Autodesk Inventor part; units mm, degrees
(part 2 of 2)
sketch "Эскиз6" plane through (0, 0, 0) normal (0, 0, -1) x (-1, 0, 0)
  line L0 (-53, 15.6179) -> (-25.3405, 4.0009) projected
  line L1 (-25.3405, 4.0009) -> (-8.0842, -5.3702) projected
  line L2 (-7.9523, -5.3473) -> (-8.0842, -5.3702) projected
  line L3 (-7.789, -5.3433) -> (-7.9523, -5.3473) projected
  line L4 (-7.444, -5.4468) -> (-7.789, -5.3433) projected
  line L5 (-6.7921, -5.8052) -> (-7.444, -5.4468) projected
  line L6 (-6.1197, -6.1235) -> (-6.7921, -5.8052) projected
  line L7 (-5.8336, -6.3424) -> (-6.1197, -6.1235) projected
  line L8 (-5.7412, -6.4771) -> (-5.8336, -6.3424) projected
  line L9 (-5.6824, -6.5974) -> (-5.7412, -6.4771) projected
  line L10 (-5.6419, -6.7101) -> (-5.6824, -6.5974) projected
  line L11 (-5.6135, -6.8178) -> (-5.6419, -6.7101) projected
  line L12 (-5.5818, -7.0232) -> (-5.6135, -6.8178) projected
  line L13 (-5.5741, -7.2193) -> (-5.5818, -7.0232) projected
  line L14 (-5.5841, -7.4089) -> (-5.5741, -7.2193) projected
  line L15 (-5.6083, -7.5933) -> (-5.5841, -7.4089) projected
  line L16 (-5.691, -7.9502) -> (-5.6083, -7.5933) projected
  line L17 (-5.802, -8.2972) -> (-5.691, -7.9502) projected
  line L18 (-5.8532, -8.6645) -> (-5.802, -8.2972) projected
  line L19 (-5.864, -9.0449) -> (-5.8532, -8.6645) projected
  line L20 (-5.8437, -9.4343) -> (-5.864, -9.0449) projected
  line L21 (-5.7962, -9.8308) -> (-5.8437, -9.4343) projected
  line L22 (-5.7233, -10.2331) -> (-5.7962, -9.8308) projected
  line L23 (-5.6263, -10.6399) -> (-5.7233, -10.2331) projected
  line L24 (-5.5062, -11.0504) -> (-5.6263, -10.6399) projected
  line L25 (-5.3633, -11.4634) -> (-5.5062, -11.0504) projected
  line L26 (-5.1983, -11.8783) -> (-5.3633, -11.4634) projected
  line L27 (-5.0602, -12.1901) -> (-5.1983, -11.8783) projected
  line L28 (-2.9375, -12.5288) -> (-5.0602, -12.1901) projected
  line L29 (-2.7092, -12.2754) -> (-2.9375, -12.5288) projected
  line L30 (-2.4233, -11.9325) -> (-2.7092, -12.2754) projected
  line L31 (-2.159, -11.5843) -> (-2.4233, -11.9325) projected
  line L32 (-1.9171, -11.2317) -> (-2.159, -11.5843) projected
  line L33 (-1.6983, -10.8752) -> (-1.9171, -11.2317) projected
  line L34 (-1.5039, -10.5156) -> (-1.6983, -10.8752) projected
  line L35 (-1.3353, -10.1535) -> (-1.5039, -10.5156) projected
  line L36 (-1.1949, -9.7897) -> (-1.3353, -10.1535) projected
  line L37 (-1.0869, -9.4249) -> (-1.1949, -9.7897) projected
  line L38 (-1.0212, -9.0599) -> (-1.0869, -9.4249) projected
  line L39 (-1.0187, -8.6955) -> (-1.0212, -9.0599) projected
  line L40 (-0.9863, -8.3307) -> (-1.0187, -8.6955) projected
  line L41 (-0.9519, -8.1479) -> (-0.9863, -8.3307) projected
  line L42 (-0.9024, -7.9646) -> (-0.9519, -8.1479) projected
  line L43 (-0.834, -7.7806) -> (-0.9024, -7.9646) projected
  line L44 (-0.74, -7.5953) -> (-0.834, -7.7806) projected
  line L45 (-0.6795, -7.5017) -> (-0.74, -7.5953) projected
  line L46 (-0.6059, -7.4072) -> (-0.6795, -7.5017) projected
  line L47 (-0.5127, -7.3112) -> (-0.6059, -7.4072) projected
  line L48 (-0.3829, -7.2119) -> (-0.5127, -7.3112) projected
  line L49 (-0.0429, -7.0929) -> (-0.3829, -7.2119) projected
  line L50 (0.6951, -6.9997) -> (-0.0429, -7.0929) projected
  line L51 (1.4262, -6.8619) -> (0.6951, -6.9997) projected
  line L52 (1.7863, -6.8709) -> (1.4262, -6.8619) projected
  line L53 (1.9402, -6.9255) -> (1.7863, -6.8709) projected
  line L54 (2.0585, -6.9883) -> (1.9402, -6.9255) projected
  line L55 (2.1575, -7.0556) -> (2.0585, -6.9883) projected
  line L56 (2.2438, -7.1261) -> (2.1575, -7.0556) projected
  line L57 (2.3901, -7.2737) -> (2.2438, -7.1261) projected
  line L58 (2.5117, -7.4278) -> (2.3901, -7.2737) projected
  line L59 (2.615, -7.5871) -> (2.5117, -7.4278) projected
  line L60 (2.7039, -7.7505) -> (2.615, -7.5871) projected
  line L61 (2.8467, -8.0877) -> (2.7039, -7.7505) projected
  line L62 (2.9609, -8.4338) -> (2.8467, -8.0877) projected
  line L63 (3.1354, -8.7611) -> (2.9609, -8.4338) projected
  line L64 (3.3502, -9.0751) -> (3.1354, -8.7611) projected
  line L65 (3.5955, -9.3782) -> (3.3502, -9.0751) projected
  line L66 (3.867, -9.6711) -> (3.5955, -9.3782) projected
  line L67 (4.1624, -9.9537) -> (3.867, -9.6711) projected
  line L68 (4.48, -10.2258) -> (4.1624, -9.9537) projected
  line L69 (4.8185, -10.4872) -> (4.48, -10.2258) projected
  line L70 (5.1768, -10.7375) -> (4.8185, -10.4872) projected
  line L71 (5.5542, -10.9761) -> (5.1768, -10.7375) projected
  line L72 (5.8492, -11.1472) -> (5.5542, -10.9761) projected
  line L73 (7.7656, -10.1735) -> (5.8492, -11.1472) projected
  line L74 (7.8013, -9.8343) -> (7.7656, -10.1735) projected
  line L75 (7.8311, -9.3888) -> (7.8013, -9.8343) projected
  line L76 (7.8403, -8.9518) -> (7.8311, -9.3888) projected
  line L77 (7.8287, -8.5243) -> (7.8403, -8.9518) projected
  line L78 (7.7961, -8.1074) -> (7.8287, -8.5243) projected
  line L79 (7.742, -7.7022) -> (7.7961, -8.1074) projected
  line L80 (7.6656, -7.3102) -> (7.742, -7.7022) projected
  line L81 (7.5654, -6.9333) -> (7.6656, -7.3102) projected
  line L82 (7.4384, -6.5746) -> (7.5654, -6.9333) projected
  line L83 (7.2769, -6.2407) -> (7.4384, -6.5746) projected
  line L84 (7.0647, -5.9445) -> (7.2769, -6.2407) projected
  line L85 (6.8765, -5.6303) -> (7.0647, -5.9445) projected
  line L86 (6.7969, -5.4622) -> (6.8765, -5.6303) projected
  line L87 (6.7292, -5.2848) -> (6.7969, -5.4622) projected
  line L88 (6.6764, -5.0958) -> (6.7292, -5.2848) projected
  line L89 (6.6435, -4.8906) -> (6.6764, -5.0958) projected
  line L90 (6.6374, -4.7793) -> (6.6435, -4.8906) projected
  line L91 (6.6415, -4.6596) -> (6.6374, -4.7793) projected
  line L92 (6.6604, -4.5271) -> (6.6415, -4.6596) projected
  line L93 (6.7071, -4.3705) -> (6.6604, -4.5271) projected
  line L94 (6.9122, -4.0744) -> (6.7071, -4.3705) projected
  line L95 (7.4545, -3.5652) -> (6.9122, -4.0744) projected
  line L96 (7.9649, -3.024) -> (7.4545, -3.5652) projected
  line L97 (8.2615, -2.8196) -> (7.9649, -3.024) projected
  line L98 (8.4182, -2.7733) -> (8.2615, -2.8196) projected
  line L99 (8.5508, -2.7546) -> (8.4182, -2.7733) projected
  line L100 (8.6705, -2.7509) -> (8.5508, -2.7546) projected
  line L101 (8.7817, -2.7571) -> (8.6705, -2.7509) projected
  line L102 (8.9868, -2.7905) -> (8.7817, -2.7571) projected
  line L103 (9.1758, -2.8438) -> (8.9868, -2.7905) projected
  line L104 (9.353, -2.9118) -> (9.1758, -2.8438) projected
  line L105 (9.5209, -2.9918) -> (9.353, -2.9118) projected
  line L106 (9.8347, -3.1808) -> (9.5209, -2.9918) projected
  line L107 (10.1304, -3.3936) -> (9.8347, -3.1808) projected
  line L108 (10.464, -3.5558) -> (10.1304, -3.3936) projected
  line L109 (10.8224, -3.6836) -> (10.464, -3.5558) projected
  line L110 (11.199, -3.7847) -> (10.8224, -3.6836) projected
  line L111 (11.5908, -3.862) -> (11.199, -3.7847) projected
  line L112 (11.9959, -3.917) -> (11.5908, -3.862) projected
  line L113 (12.4128, -3.9505) -> (11.9959, -3.917) projected
  line L114 (12.8403, -3.963) -> (12.4128, -3.9505) projected
  line L115 (13.2773, -3.9548) -> (12.8403, -3.963) projected
  line L116 (13.7228, -3.9261) -> (13.2773, -3.9548) projected
  line L117 (14.0621, -3.891) -> (13.7228, -3.9261) projected
  line L118 (15.0401, -1.9769) -> (14.0621, -3.891) projected
  line L119 (14.8697, -1.6815) -> (15.0401, -1.9769) projected
  line L120 (14.6319, -1.3036) -> (14.8697, -1.6815) projected
  line L121 (14.3824, -0.9447) -> (14.6319, -1.3036) projected
  line L122 (14.1218, -0.6056) -> (14.3824, -0.9447) projected
  line L123 (13.8504, -0.2874) -> (14.1218, -0.6056) projected
  line L124 (13.5684, 0.0086) -> (13.8504, -0.2874) projected
  line L125 (13.2762, 0.2808) -> (13.5684, 0.0086) projected
  line L126 (12.9736, 0.5268) -> (13.2762, 0.2808) projected
  line L127 (12.66, 0.7423) -> (12.9736, 0.5268) projected
  line L128 (12.3332, 0.9175) -> (12.66, 0.7423) projected
  line L129 (11.9874, 1.0325) -> (12.3332, 0.9175) projected
  line L130 (11.6504, 1.1761) -> (11.9874, 1.0325) projected
  line L131 (11.4872, 1.2653) -> (11.6504, 1.1761) projected
  line L132 (11.3282, 1.369) -> (11.4872, 1.2653) projected
  line L133 (11.1743, 1.4909) -> (11.3282, 1.369) projected
  line L134 (11.0271, 1.6375) -> (11.1743, 1.4909) projected
  line L135 (10.9568, 1.724) -> (11.0271, 1.6375) projected
  line L136 (10.8897, 1.8232) -> (10.9568, 1.724) projected
  line L137 (10.8272, 1.9416) -> (10.8897, 1.8232) projected
  line L138 (10.7729, 2.0956) -> (10.8272, 1.9416) projected
  line L139 (10.7647, 2.4558) -> (10.7729, 2.0956) projected
  line L140 (10.9042, 3.1865) -> (10.7647, 2.4558) projected
  line L141 (10.999, 3.9243) -> (10.9042, 3.1865) projected
  line L142 (11.1188, 4.264) -> (10.999, 3.9243) projected
  line L143 (11.2183, 4.3936) -> (11.1188, 4.264) projected
  line L144 (11.3146, 4.4866) -> (11.2183, 4.3936) projected
  line L145 (11.4093, 4.56) -> (11.3146, 4.4866) projected
  line L146 (11.5029, 4.6203) -> (11.4093, 4.56) projected
  line L147 (11.6885, 4.7139) -> (11.5029, 4.6203) projected
  line L148 (11.8727, 4.7818) -> (11.6885, 4.7139) projected
  line L149 (12.056, 4.8309) -> (11.8727, 4.7818) projected
  line L150 (12.2389, 4.8649) -> (12.056, 4.8309) projected
  line L151 (12.6038, 4.8965) -> (12.2389, 4.8649) projected
  line L152 (12.9682, 4.8982) -> (12.6038, 4.8965) projected
  line L153 (13.3334, 4.963) -> (12.9682, 4.8982) projected
  line L154 (13.6984, 5.0703) -> (13.3334, 4.963) projected
  line L155 (14.0625, 5.2099) -> (13.6984, 5.0703) projected
  line L156 (14.425, 5.3776) -> (14.0625, 5.2099) projected
  line L157 (14.785, 5.5713) -> (14.425, 5.3776) projected
  line L158 (15.142, 5.7892) -> (14.785, 5.5713) projected
  line L159 (15.4952, 6.0303) -> (15.142, 5.7892) projected
  line L160 (15.8439, 6.2938) -> (15.4952, 6.0303) projected
  line L161 (16.1875, 6.579) -> (15.8439, 6.2938) projected
  line L162 (16.4414, 6.8067) -> (16.1875, 6.579) projected
  line L163 (16.1075, 8.9301) -> (16.4414, 6.8067) projected
  line L164 (15.796, 9.069) -> (16.1075, 8.9301) projected
  line L165 (15.3815, 9.2349) -> (15.796, 9.069) projected
  line L166 (14.9687, 9.3787) -> (15.3815, 9.2349) projected
  line L167 (14.5586, 9.4998) -> (14.9687, 9.3787) projected
  line L168 (14.1519, 9.5976) -> (14.5586, 9.4998) projected
  line L169 (13.7498, 9.6714) -> (14.1519, 9.5976) projected
  line L170 (13.3534, 9.7199) -> (13.7498, 9.6714) projected
  line L171 (12.964, 9.741) -> (13.3534, 9.7199) projected
  line L172 (12.5837, 9.731) -> (12.964, 9.741) projected
  line L173 (12.2162, 9.6807) -> (12.5837, 9.731) projected
  line L174 (11.8689, 9.5704) -> (12.2162, 9.6807) projected
  line L175 (11.5119, 9.4885) -> (11.8689, 9.5704) projected
  line L176 (11.3274, 9.4648) -> (11.5119, 9.4885) projected
  line L177 (11.1379, 9.4552) -> (11.3274, 9.4648) projected
  line L178 (10.9417, 9.4634) -> (11.1379, 9.4552) projected
  line L179 (10.7364, 9.4955) -> (10.9417, 9.4634) projected
  line L180 (10.6287, 9.5241) -> (10.7364, 9.4955) projected
  line L181 (10.5161, 9.5649) -> (10.6287, 9.5241) projected
  line L182 (10.3959, 9.6239) -> (10.5161, 9.5649) projected
  line L183 (10.2615, 9.7167) -> (10.3959, 9.6239) projected
  line L184 (10.0432, 10.0032) -> (10.2615, 9.7167) projected
  line L185 (9.7265, 10.6764) -> (10.0432, 10.0032) projected
  line L186 (9.3696, 11.329) -> (9.7265, 10.6764) projected
  line L187 (9.2668, 11.6743) -> (9.3696, 11.329) projected
  line L188 (9.2712, 11.8376) -> (9.2668, 11.6743) projected
  line L189 (9.2943, 11.9695) -> (9.2712, 11.8376) projected
  line L190 (9.3278, 12.0845) -> (9.2943, 11.9695) projected
  line L191 (9.3681, 12.1883) -> (9.3278, 12.0845) projected
  line L192 (9.4633, 12.3731) -> (9.3681, 12.1883) projected
  line L193 (9.5723, 12.5363) -> (9.4633, 12.3731) projected
  line L194 (9.6918, 12.6838) -> (9.5723, 12.5363) projected
  line L195 (9.8198, 12.8188) -> (9.6918, 12.6838) projected
  line L196 (10.0964, 13.0589) -> (9.8198, 12.8188) projected
  line L197 (10.3902, 13.2744) -> (10.0964, 13.0589) projected
  line L198 (10.6476, 13.5415) -> (10.3902, 13.2744) projected
  line L199 (10.8798, 13.8428) -> (10.6476, 13.5415) projected
  line L200 (11.0924, 14.1698) -> (10.8798, 13.8428) projected
  line L201 (11.1891, 14.3431) -> (11.0924, 14.1698) projected
  arc A0 (11.1891, 14.3431) -> (-16.1963, 14.3431) centre (-2.5036, -3.8906) ccw projected
  arc A1 (-25.3405, 9.161) -> (-16.1963, 14.3431) centre (-40.8164, 47.1281) ccw projected
  line L202 (-25.3405, 9.161) -> (-53, 20.778) projected
  line L203 (-53, 20.778) -> (-57, 20.778) projected
  line L204 (-57, 20.778) -> (-57, 17.5182) projected
  line L205 (-57, 17.5182) -> (-76.2555, 1.8259) projected
  line L206 (-76.2555, 1.8259) -> (-73.7286, -1.2748) projected
  line L207 (-73.7286, -1.2748) -> (-57, 12.3581) projected
  line L208 (-57, 12.3581) -> (-57, -9) projected
  line L209 (-57, -9) -> (-53, -9) projected
  line L210 (-53, -9) -> (-53, 15.6179) projected
  circle A2 centre (-8.3767, 1.5633) radius 1.6 projected
  circle A3 centre (2.3455, -2.0471) radius 1.6 projected
  circle A4 centre (5.9559, 8.675) radius 1.6 projected
  circle A5 centre (-4.7663, 12.2855) radius 1.6 projected
  circle A6 centre (-1.2104, 5.1192) radius 2.5 projected
  line L211 (-57, 17.5182) -> (-57, 12.3581)
  point P0 (0, 0)
  constraints: 2 end point, 1 collinear
extrude "Выдавливание6" cut sketch "Эскиз6" against normal blind 10 contours L207 L206 L205 L211
sketch "Эскиз7" plane through (0, 0, 5) normal (0, 0, 1) x (1, 0, 0)
  line L0 (39.5581, 1.9289) -> (53.904, -11.9897) projected
  line L1 (39.5581, 1.9289) -> (53.904, -11.9897) construction
  line L2 (71.9316, -0.8693) -> (40.2367, -32.4918) construction
  line L3 (71.9316, -0.8693) -> (71.9317, -0.7909) construction
  line L4 (71.9317, -0.7909) -> (40.1893, -0.7429) construction
  line L5 (40.1893, -0.7429) -> (40.1583, -32.5308) construction
  ellipse E0 centre (40.323, 96.1032) end of major axis (40.1583, -32.5308) minor radius 3.174 (40.1583, -32.5308) -> (40.2367, -32.4918) ccw construction
  line L6 (71.9495, -32.6204) -> (72.0099, -0.8302) construction
  ellipse E1 centre (71.7261, -129.4732) end of major axis (71.4423, -258.1162) minor radius 3.1711 (72.0099, -0.8302) -> (71.9316, -0.8693) ccw construction
  line L7 (71.9316, -0.8693) -> (40.2367, -32.4918) construction
  line L8 (40.2367, -32.4918) -> (40.2366, -32.5701) construction
  line L9 (40.2366, -32.5701) -> (71.9495, -32.6204) construction
  line L10 (61.1948, -58.9491) -> (61.3584, -29.5225) projected
  line L11 (61.3584, -29.5225) -> (54.845, -29.4863) projected
  line L12 (54.845, -29.4863) -> (43.8928, -40.4135) projected
  line L13 (43.8928, -40.4135) -> (39.1927, -45.5003) projected
  line L14 (39.1927, -45.5003) -> (23.9385, -36.7753) projected
  line L15 (9.9184, -17.7195) -> (23.9385, -36.7753) projected
  line L16 (9.9184, -17.7195) -> (9.6501, -17.5929) projected
  line L17 (9.4478, -17.7158) -> (9.6501, -17.5929) projected
  line L18 (9.1396, -17.9389) -> (9.4478, -17.7158) projected
  line L19 (8.8648, -18.188) -> (9.1396, -17.9389) projected
  line L20 (8.6405, -18.4751) -> (8.8648, -18.188) projected
  line L21 (8.3922, -18.7444) -> (8.6405, -18.4751) projected
  line L22 (8.2533, -18.8682) -> (8.3922, -18.7444) projected
  line L23 (8.1023, -18.9831) -> (8.2533, -18.8682) projected
  line L24 (7.9358, -19.0872) -> (8.1023, -18.9831) projected
  line L25 (7.7483, -19.1767) -> (7.9358, -19.0872) projected
  line L26 (7.6432, -19.2139) -> (7.7483, -19.1767) projected
  line L27 (7.5273, -19.2438) -> (7.6432, -19.2139) projected
  line L28 (7.3948, -19.263) -> (7.5273, -19.2438) projected
  line L29 (7.2314, -19.2624) -> (7.3948, -19.263) projected
  line L30 (6.8894, -19.1492) -> (7.2314, -19.2624) projected
  line L31 (6.2479, -18.7726) -> (6.8894, -19.1492) projected
  line L32 (5.5847, -18.4357) -> (6.2479, -18.7726) projected
  line L33 (5.3049, -18.2088) -> (5.5847, -18.4357) projected
  line L34 (5.2162, -18.0716) -> (5.3049, -18.2088) projected
  line L35 (5.1609, -17.9496) -> (5.2162, -18.0716) projected
  line L36 (5.1235, -17.8359) -> (5.1609, -17.9496) projected
  line L37 (5.0982, -17.7274) -> (5.1235, -17.8359) projected
  line L38 (5.0723, -17.5212) -> (5.0982, -17.7274) projected
  line L39 (5.0701, -17.3249) -> (5.0723, -17.5212) projected
  line L40 (5.0854, -17.1357) -> (5.0701, -17.3249) projected
  line L41 (5.1147, -16.952) -> (5.0854, -17.1357) projected
  line L42 (5.2074, -16.5976) -> (5.1147, -16.952) projected
  line L43 (5.3282, -16.2538) -> (5.2074, -16.5976) projected
  line L44 (5.3896, -15.8881) -> (5.3282, -16.2538) projected
  line L45 (5.4111, -15.5082) -> (5.3896, -15.8881) projected
  line L46 (5.4018, -15.1184) -> (5.4111, -15.5082) projected
  line L47 (5.3654, -14.7206) -> (5.4018, -15.1184) projected
  line L48 (5.3039, -14.3165) -> (5.3654, -14.7206) projected
  line L49 (5.2184, -13.9071) -> (5.3039, -14.3165) projected
  line L50 (5.1098, -13.4935) -> (5.2184, -13.9071) projected
  line L51 (4.9786, -13.0765) -> (5.1098, -13.4935) projected
  line L52 (4.8253, -12.6572) -> (4.9786, -13.0765) projected
  line L53 (4.696, -12.3416) -> (4.8253, -12.6572) projected
  line L54 (2.5836, -11.9435) -> (4.696, -12.3416) projected
  line L55 (2.3483, -12.1904) -> (2.5836, -11.9435) projected
  line L56 (2.0529, -12.5251) -> (2.3483, -12.1904) projected
  line L57 (1.7789, -12.8657) -> (2.0529, -12.5251) projected
  line L58 (1.5272, -13.2114) -> (1.7789, -12.8657) projected
  line L59 (1.2985, -13.5616) -> (1.5272, -13.2114) projected
  line L60 (1.0941, -13.9156) -> (1.2985, -13.5616) projected
  line L61 (0.9154, -14.2728) -> (1.0941, -13.9156) projected
  line L62 (0.7648, -14.6325) -> (0.9154, -14.2728) projected
  line L63 (0.6465, -14.9941) -> (0.7648, -14.6325) projected
  line L64 (0.5707, -15.3572) -> (0.6465, -14.9941) projected
  line L65 (0.558, -15.7213) -> (0.5707, -15.3572) projected
  line L66 (0.5153, -16.0851) -> (0.558, -15.7213) projected
  line L67 (0.4758, -16.2669) -> (0.5153, -16.0851) projected
  line L68 (0.4212, -16.4487) -> (0.4758, -16.2669) projected
  line L69 (0.3476, -16.6307) -> (0.4212, -16.4487) projected
  line L70 (0.2485, -16.8133) -> (0.3476, -16.6307) projected
  line L71 (0.1854, -16.9051) -> (0.2485, -16.8133) projected
  line L72 (0.1092, -16.9975) -> (0.1854, -16.9051) projected
  line L73 (0.0132, -17.0909) -> (0.1092, -16.9975) projected
  line L74 (-0.1193, -17.1865) -> (0.0132, -17.0909) projected
  line L75 (-0.4625, -17.2959) -> (-0.1193, -17.1865) projected
  line L76 (-1.2028, -17.3684) -> (-0.4625, -17.2959) projected
  line L77 (-1.9374, -17.4856) -> (-1.2028, -17.3684) projected
  line L78 (-2.2972, -17.4665) -> (-1.9374, -17.4856) projected
  line L79 (-2.4495, -17.4076) -> (-2.2972, -17.4665) projected
  line L80 (-2.566, -17.3415) -> (-2.4495, -17.4076) projected
  line L81 (-2.6631, -17.2714) -> (-2.566, -17.3415) projected
  line L82 (-2.7474, -17.1985) -> (-2.6631, -17.2714) projected
  line L83 (-2.8895, -17.0469) -> (-2.7474, -17.1985) projected
  line L84 (-3.0066, -16.8894) -> (-2.8895, -17.0469) projected
  line L85 (-3.1055, -16.7273) -> (-3.0066, -16.8894) projected
  line L86 (-3.1897, -16.5615) -> (-3.1055, -16.7273) projected
  line L87 (-3.323, -16.2203) -> (-3.1897, -16.5615) projected
  line L88 (-3.4274, -15.8712) -> (-3.323, -16.2203) projected
  line L89 (-3.5927, -15.5392) -> (-3.4274, -15.8712) projected
  line L90 (-3.7986, -15.2192) -> (-3.5927, -15.5392) projected
  line L91 (-4.0352, -14.9093) -> (-3.7986, -15.2192) projected
  line L92 (-4.2985, -14.6089) -> (-4.0352, -14.9093) projected
  line L93 (-4.5858, -14.3182) -> (-4.2985, -14.6089) projected
  line L94 (-4.8956, -14.0372) -> (-4.5858, -14.3182) projected
  line L95 (-5.2266, -13.7664) -> (-4.8956, -14.0372) projected
  line L96 (-5.5778, -13.5062) -> (-5.2266, -13.7664) projected
  line L97 (-5.9483, -13.2571) -> (-5.5778, -13.5062) projected
  line L98 (-6.2384, -13.0778) -> (-5.9483, -13.2571) projected
  line L99 (-8.1813, -13.9973) -> (-6.2384, -13.0778) projected
  line L100 (-8.2266, -14.3353) -> (-8.1813, -13.9973) projected
  line L101 (-8.2689, -14.7798) -> (-8.2266, -14.3353) projected
  line L102 (-8.2903, -15.2163) -> (-8.2689, -14.7798) projected
  line L103 (-8.2908, -15.644) -> (-8.2903, -15.2163) projected
  line L104 (-8.2699, -16.0617) -> (-8.2908, -15.644) projected
  line L105 (-8.2272, -16.4683) -> (-8.2699, -16.0617) projected
  line L106 (-8.1619, -16.8623) -> (-8.2272, -16.4683) projected
  line L107 (-8.0722, -17.2418) -> (-8.1619, -16.8623) projected
  line L108 (-7.9554, -17.6039) -> (-8.0722, -17.2418) projected
  line L109 (-7.8034, -17.9422) -> (-7.9554, -17.6039) projected
  line L110 (-7.5996, -18.2443) -> (-7.8034, -17.9422) projected
  line L111 (-7.4203, -18.5636) -> (-7.5996, -18.2443) projected
  line L112 (-7.3454, -18.7339) -> (-7.4203, -18.5636) projected
  line L113 (-7.2827, -18.9131) -> (-7.3454, -18.7339) projected
  line L114 (-7.2352, -19.1036) -> (-7.2827, -18.9131) projected
  line L115 (-7.2081, -19.3096) -> (-7.2352, -19.1036) projected
  line L116 (-7.2052, -19.421) -> (-7.2081, -19.3096) projected
  line L117 (-7.2126, -19.5405) -> (-7.2052, -19.421) projected
  line L118 (-7.2353, -19.6725) -> (-7.2126, -19.5405) projected
  line L119 (-7.2863, -19.8277) -> (-7.2353, -19.6725) projected
  line L120 (-7.4996, -20.1179) -> (-7.2863, -19.8277) projected
  line L121 (-8.056, -20.6117) -> (-7.4996, -20.1179) projected
  line L122 (-8.5814, -21.1383) -> (-8.056, -20.6117) projected
  line L123 (-8.8836, -21.3343) -> (-8.5814, -21.1383) projected
  line L124 (-9.0415, -21.3762) -> (-8.8836, -21.3343) projected
  line L125 (-9.1746, -21.3912) -> (-9.0415, -21.3762) projected
  line L126 (-9.2944, -21.3915) -> (-9.1746, -21.3912) projected
  line L127 (-9.4054, -21.3821) -> (-9.2944, -21.3915) projected
  line L128 (-9.6095, -21.343) -> (-9.4054, -21.3821) projected
  line L129 (-9.7969, -21.2845) -> (-9.6095, -21.343) projected
  line L130 (-9.9721, -21.2114) -> (-9.7969, -21.2845) projected
  line L131 (-10.1377, -21.1268) -> (-9.9721, -21.2114) projected
  line L132 (-10.4461, -20.9291) -> (-10.1377, -21.1268) projected
  line L133 (-10.7357, -20.708) -> (-10.4461, -20.9291) projected
  line L134 (-11.0646, -20.5366) -> (-10.7357, -20.708) projected
  line L135 (-11.4192, -20.3987) -> (-11.0646, -20.5366) projected
  line L136 (-11.7929, -20.2871) -> (-11.4192, -20.3987) projected
  line L137 (-12.1824, -20.1988) -> (-11.7929, -20.2871) projected
  line L138 (-12.5858, -20.1325) -> (-12.1824, -20.1988) projected
  line L139 (-13.0015, -20.0873) -> (-12.5858, -20.1325) projected
  line L140 (-13.4285, -20.0628) -> (-13.0015, -20.0873) projected
  line L141 (-13.8655, -20.0587) -> (-13.4285, -20.0628) projected
  line L142 (-14.3117, -20.0749) -> (-13.8655, -20.0587) projected
  line L143 (-14.6518, -20.1004) -> (-14.3117, -20.0749) projected
  line L144 (-15.6832, -21.9863) -> (-14.6518, -20.1004) projected
  line L145 (-15.5212, -22.2864) -> (-15.6832, -21.9863) projected
  line L146 (-15.2941, -22.6708) -> (-15.5212, -22.2864) projected
  line L147 (-15.0548, -23.0366) -> (-15.2941, -22.6708) projected
  line L148 (-14.8038, -23.3828) -> (-15.0548, -23.0366) projected
  line L149 (-14.5414, -23.7085) -> (-14.8038, -23.3828) projected
  line L150 (-14.2679, -24.0123) -> (-14.5414, -23.7085) projected
  line L151 (-13.9834, -24.2927) -> (-14.2679, -24.0123) projected
  line L152 (-13.6879, -24.547) -> (-13.9834, -24.2927) projected
  line L153 (-13.3805, -24.7713) -> (-13.6879, -24.547) projected
  line L154 (-13.0587, -24.9556) -> (-13.3805, -24.7713) projected
  line L155 (-12.7162, -25.0802) -> (-13.0587, -24.9556) projected
  line L156 (-12.3834, -25.2332) -> (-12.7162, -25.0802) projected
  line L157 (-12.2228, -25.327) -> (-12.3834, -25.2332) projected
  line L158 (-12.0668, -25.4351) -> (-12.2228, -25.327) projected
  line L159 (-11.9164, -25.5613) -> (-12.0668, -25.4351) projected
  line L160 (-11.7733, -25.712) -> (-11.9164, -25.5613) projected
  line L161 (-11.7055, -25.8004) -> (-11.7733, -25.712) projected
  line L162 (-11.6412, -25.9014) -> (-11.7055, -25.8004) projected
  line L163 (-11.582, -26.0215) -> (-11.6412, -25.9014) projected
  line L164 (-11.5321, -26.1771) -> (-11.582, -26.0215) projected
  line L165 (-11.5341, -26.5373) -> (-11.5321, -26.1771) projected
  line L166 (-11.6939, -27.2638) -> (-11.5341, -26.5373) projected
  line L167 (-11.8095, -27.9987) -> (-11.6939, -27.2638) projected
  line L168 (-11.9388, -28.3349) -> (-11.8095, -27.9987) projected
  line L169 (-12.0419, -28.4616) -> (-11.9388, -28.3349) projected
  line L170 (-12.1407, -28.5519) -> (-12.0419, -28.4616) projected
  line L171 (-12.2374, -28.6226) -> (-12.1407, -28.5519) projected
  line L172 (-12.3328, -28.6803) -> (-12.2374, -28.6226) projected
  line L173 (-12.5209, -28.7686) -> (-12.3328, -28.6803) projected
  line L174 (-12.7069, -28.8313) -> (-12.5209, -28.7686) projected
  line L175 (-12.8916, -28.8752) -> (-12.7069, -28.8313) projected
  line L176 (-13.0753, -28.9041) -> (-12.8916, -28.8752) projected
  line L177 (-13.441, -28.9254) -> (-13.0753, -28.9041) projected
  line L178 (-13.8052, -28.9168) -> (-13.441, -28.9254) projected
  line L179 (-14.1721, -28.9714) -> (-13.8052, -28.9168) projected
  line L180 (-14.54, -29.0684) -> (-14.1721, -28.9714) projected
  line L181 (-14.9079, -29.1977) -> (-14.54, -29.0684) projected
  line L182 (-15.2749, -29.3552) -> (-14.9079, -29.1977) projected
  line L183 (-15.6403, -29.5386) -> (-15.2749, -29.3552) projected
  line L184 (-16.0032, -29.7465) -> (-15.6403, -29.5386) projected
  line L185 (-16.363, -29.9776) -> (-16.0032, -29.7465) projected
  line L186 (-16.5142, -30.0852) -> (-16.363, -29.9776) projected
  arc A0 (-16.5142, -30.0852) -> (11.3827, -43.2543) centre (4.6035, -21.4828) ccw projected
  arc A1 (21.7357, -41.4416) -> (11.3827, -43.2543) centre (23.572, -82.4005) ccw projected
  line L187 (21.7357, -41.4416) -> (51.8609, -57.1396) projected
  line L188 (51.8609, -57.1396) -> (57.3573, -59.8994) projected
  line L189 (57.3573, -59.8994) -> (61.1948, -58.9491) projected
  circle A2 centre (1.3062, -37.48) radius 1.6 projected
  circle A3 centre (8.3056, -28.5914) radius 1.6 projected
  circle A4 centre (-0.583, -21.5919) radius 1.6 projected
  circle A5 centre (0.3616, -29.536) radius 2.5 projected
  circle A6 centre (-7.5825, -30.4806) radius 1.6 projected
  line L190 (40.1738, -16.6369) -> (71.9797, -16.7253)
  ellipse E2 centre (39.6963, -129.376) end of major axis (40.2467, -0.7431) minor radius 3.174 (40.3248, -0.7826) -> (40.2467, -0.7431) ccw construction
  line L191 (40.3248, -0.7826) -> (40.3251, -0.7042) construction
  line L192 (61.4297, 25.5578) -> (61.4297, -3.8692)
  line L193 (61.4297, -3.8692) -> (54.9162, -3.8692)
  line L194 (54.9162, -3.8692) -> (44.0249, 7.1187)
  line L195 (44.0249, 7.1187) -> (40.9018, 10.5367)
  line L196 (52.0859, 23.8002) -> (57.5975, 26.5294)
  line L197 (57.5975, 26.5294) -> (61.4297, 25.5578)
  line L198 (53, 15.6179) -> (25.3405, 4.0009) projected
  circle A7 centre (8.3767, 1.5633) radius 1.6 projected
  circle A8 centre (-2.3455, -2.0471) radius 1.6 projected
  circle A9 centre (-5.9559, 8.675) radius 1.6 projected
  circle A10 centre (4.7663, 12.2855) radius 1.6 projected
  circle A11 centre (1.2104, 5.1192) radius 2.5 projected
  line L199 (57, -9) -> (57, 20.778) projected
  line L200 (53, 20.778) -> (57, 20.778) projected
  line L201 (25.3405, 9.161) -> (53, 20.778) projected
  arc A12 (16.1963, 14.3431) -> (25.3405, 9.161) centre (40.8164, 47.1281) ccw projected
  arc A13 (16.1963, 14.3431) -> (-11.1891, 14.3431) centre (2.5036, -3.8906) ccw projected
  line L202 (-11.1891, 14.3431) -> (-11.0924, 14.1698) projected
  line L203 (-11.0924, 14.1698) -> (-10.8798, 13.8428) projected
  line L204 (-10.8798, 13.8428) -> (-10.6476, 13.5415) projected
  line L205 (-10.6476, 13.5415) -> (-10.3902, 13.2744) projected
  line L206 (-10.3902, 13.2744) -> (-10.0964, 13.0589) projected
  line L207 (-10.0964, 13.0589) -> (-9.8198, 12.8188) projected
  line L208 (-9.8198, 12.8188) -> (-9.6918, 12.6838) projected
  line L209 (-9.6918, 12.6838) -> (-9.5723, 12.5363) projected
  line L210 (-9.5723, 12.5363) -> (-9.4633, 12.3731) projected
  line L211 (-9.4633, 12.3731) -> (-9.3681, 12.1883) projected
  line L212 (-9.3681, 12.1883) -> (-9.3278, 12.0845) projected
  line L213 (-9.3278, 12.0845) -> (-9.2943, 11.9695) projected
  line L214 (-9.2943, 11.9695) -> (-9.2712, 11.8376) projected
  line L215 (-9.2712, 11.8376) -> (-9.2668, 11.6743) projected
  line L216 (-9.2668, 11.6743) -> (-9.3696, 11.329) projected
  line L217 (-9.3696, 11.329) -> (-9.7265, 10.6764) projected
  line L218 (-9.7265, 10.6764) -> (-10.0432, 10.0032) projected
  line L219 (-10.0432, 10.0032) -> (-10.2615, 9.7167) projected
  line L220 (-10.2615, 9.7167) -> (-10.3959, 9.6239) projected
  line L221 (-10.3959, 9.6239) -> (-10.5161, 9.5649) projected
  line L222 (-10.5161, 9.5649) -> (-10.6287, 9.5241) projected
  line L223 (-10.6287, 9.5241) -> (-10.7364, 9.4955) projected
  line L224 (-10.7364, 9.4955) -> (-10.9417, 9.4634) projected
  line L225 (-10.9417, 9.4634) -> (-11.1379, 9.4552) projected
  line L226 (-11.1379, 9.4552) -> (-11.3274, 9.4648) projected
  line L227 (-11.3274, 9.4648) -> (-11.5119, 9.4885) projected
  line L228 (-11.5119, 9.4885) -> (-11.8689, 9.5704) projected
  line L229 (-11.8689, 9.5704) -> (-12.2162, 9.6807) projected
  line L230 (-12.2162, 9.6807) -> (-12.5837, 9.731) projected
  line L231 (-12.5837, 9.731) -> (-12.964, 9.741) projected
  line L232 (-12.964, 9.741) -> (-13.3534, 9.7199) projected
  line L233 (-13.3534, 9.7199) -> (-13.7498, 9.6714) projected
  line L234 (-13.7498, 9.6714) -> (-14.1519, 9.5976) projected
  line L235 (-14.1519, 9.5976) -> (-14.5586, 9.4998) projected
  line L236 (-14.5586, 9.4998) -> (-14.9687, 9.3787) projected
  line L237 (-14.9687, 9.3787) -> (-15.3815, 9.2349) projected
  line L238 (-15.3815, 9.2349) -> (-15.796, 9.069) projected
  line L239 (-15.796, 9.069) -> (-16.1075, 8.9301) projected
  line L240 (-16.1075, 8.9301) -> (-16.4414, 6.8067) projected
  line L241 (-16.4414, 6.8067) -> (-16.1875, 6.579) projected
  line L242 (-16.1875, 6.579) -> (-15.8439, 6.2938) projected
  line L243 (-15.8439, 6.2938) -> (-15.4952, 6.0303) projected
  line L244 (-15.4952, 6.0303) -> (-15.142, 5.7892) projected
  line L245 (-15.142, 5.7892) -> (-14.785, 5.5713) projected
  line L246 (-14.785, 5.5713) -> (-14.425, 5.3776) projected
  line L247 (-14.425, 5.3776) -> (-14.0625, 5.2099) projected
  line L248 (-14.0625, 5.2099) -> (-13.6984, 5.0703) projected
  line L249 (-13.6984, 5.0703) -> (-13.3334, 4.963) projected
  line L250 (-13.3334, 4.963) -> (-12.9682, 4.8982) projected
  line L251 (-12.9682, 4.8982) -> (-12.6038, 4.8965) projected
  line L252 (-12.6038, 4.8965) -> (-12.2389, 4.8649) projected
  line L253 (-12.2389, 4.8649) -> (-12.056, 4.8309) projected
  line L254 (-12.056, 4.8309) -> (-11.8727, 4.7818) projected
  line L255 (-11.8727, 4.7818) -> (-11.6885, 4.7139) projected
  line L256 (-11.6885, 4.7139) -> (-11.5029, 4.6203) projected
  line L257 (-11.5029, 4.6203) -> (-11.4093, 4.56) projected
  line L258 (-11.4093, 4.56) -> (-11.3146, 4.4866) projected
  line L259 (-11.3146, 4.4866) -> (-11.2183, 4.3936) projected
  line L260 (-11.2183, 4.3936) -> (-11.1188, 4.264) projected
  line L261 (-11.1188, 4.264) -> (-10.999, 3.9243) projected
  line L262 (-10.999, 3.9243) -> (-10.9042, 3.1865) projected
  line L263 (-10.9042, 3.1865) -> (-10.7647, 2.4558) projected
  line L264 (-10.7647, 2.4558) -> (-10.7729, 2.0956) projected
  line L265 (-10.7729, 2.0956) -> (-10.8272, 1.9416) projected
  line L266 (-10.8272, 1.9416) -> (-10.8897, 1.8232) projected
  line L267 (-10.8897, 1.8232) -> (-10.9568, 1.724) projected
  line L268 (-10.9568, 1.724) -> (-11.0271, 1.6375) projected
  line L269 (-11.0271, 1.6375) -> (-11.1743, 1.4909) projected
  line L270 (-11.1743, 1.4909) -> (-11.3282, 1.369) projected
  line L271 (-11.3282, 1.369) -> (-11.4872, 1.2653) projected
  line L272 (-11.4872, 1.2653) -> (-11.6504, 1.1761) projected
  line L273 (-11.6504, 1.1761) -> (-11.9874, 1.0325) projected
  line L274 (-11.9874, 1.0325) -> (-12.3332, 0.9175) projected
  line L275 (-12.3332, 0.9175) -> (-12.66, 0.7423) projected
  line L276 (-12.66, 0.7423) -> (-12.9736, 0.5268) projected
  line L277 (-12.9736, 0.5268) -> (-13.2762, 0.2808) projected
  line L278 (-13.2762, 0.2808) -> (-13.5684, 0.0086) projected
  line L279 (-13.5684, 0.0086) -> (-13.8504, -0.2874) projected
  line L280 (-13.8504, -0.2874) -> (-14.1218, -0.6056) projected
  line L281 (-14.1218, -0.6056) -> (-14.3824, -0.9447) projected
  line L282 (-14.3824, -0.9447) -> (-14.6319, -1.3036) projected
  line L283 (-14.6319, -1.3036) -> (-14.8697, -1.6815) projected
  line L284 (-14.8697, -1.6815) -> (-15.0401, -1.9769) projected
  line L285 (-15.0401, -1.9769) -> (-14.0621, -3.891) projected
  line L286 (-14.0621, -3.891) -> (-13.7228, -3.9261) projected
  line L287 (-13.7228, -3.9261) -> (-13.2773, -3.9548) projected
  line L288 (-13.2773, -3.9548) -> (-12.8403, -3.963) projected
  line L289 (-12.8403, -3.963) -> (-12.4128, -3.9505) projected
  line L290 (-12.4128, -3.9505) -> (-11.9959, -3.917) projected
  line L291 (-11.9959, -3.917) -> (-11.5908, -3.862) projected
  line L292 (-11.5908, -3.862) -> (-11.199, -3.7847) projected
  line L293 (-11.199, -3.7847) -> (-10.8224, -3.6836) projected
  line L294 (-10.8224, -3.6836) -> (-10.464, -3.5558) projected
  line L295 (-10.464, -3.5558) -> (-10.1304, -3.3936) projected
  line L296 (-10.1304, -3.3936) -> (-9.8347, -3.1808) projected
  line L297 (-9.8347, -3.1808) -> (-9.5209, -2.9918) projected
  line L298 (-9.5209, -2.9918) -> (-9.353, -2.9118) projected
  line L299 (-9.353, -2.9118) -> (-9.1758, -2.8438) projected
  line L300 (-9.1758, -2.8438) -> (-8.9868, -2.7905) projected
  line L301 (-8.9868, -2.7905) -> (-8.7817, -2.7571) projected
  line L302 (-8.7817, -2.7571) -> (-8.6705, -2.7509) projected
  line L303 (-8.6705, -2.7509) -> (-8.5508, -2.7546) projected
  line L304 (-8.5508, -2.7546) -> (-8.4182, -2.7733) projected
  line L305 (-8.4182, -2.7733) -> (-8.2615, -2.8196) projected
  line L306 (-8.2615, -2.8196) -> (-7.9649, -3.024) projected
  line L307 (-7.9649, -3.024) -> (-7.4545, -3.5652) projected
  line L308 (-7.4545, -3.5652) -> (-6.9122, -4.0744) projected
  line L309 (-6.9122, -4.0744) -> (-6.7071, -4.3705) projected
  line L310 (-6.7071, -4.3705) -> (-6.6604, -4.5271) projected
  line L311 (-6.6604, -4.5271) -> (-6.6415, -4.6596) projected
  line L312 (-6.6415, -4.6596) -> (-6.6374, -4.7793) projected
  line L313 (-6.6374, -4.7793) -> (-6.6435, -4.8906) projected
  line L314 (-6.6435, -4.8906) -> (-6.6764, -5.0958) projected
  line L315 (-6.6764, -5.0958) -> (-6.7292, -5.2848) projected
  line L316 (-6.7292, -5.2848) -> (-6.7969, -5.4622) projected
  line L317 (-6.7969, -5.4622) -> (-6.8765, -5.6303) projected
  line L318 (-6.8765, -5.6303) -> (-7.0647, -5.9445) projected
  line L319 (-7.0647, -5.9445) -> (-7.2769, -6.2407) projected
  line L320 (-7.2769, -6.2407) -> (-7.4384, -6.5746) projected
  line L321 (-7.4384, -6.5746) -> (-7.5654, -6.9333) projected
  line L322 (-7.5654, -6.9333) -> (-7.6656, -7.3102) projected
  line L323 (-7.6656, -7.3102) -> (-7.742, -7.7022) projected
  line L324 (-7.742, -7.7022) -> (-7.7961, -8.1074) projected
  line L325 (-7.7961, -8.1074) -> (-7.8287, -8.5243) projected
  line L326 (-7.8287, -8.5243) -> (-7.8403, -8.9518) projected
  line L327 (-7.8403, -8.9518) -> (-7.8311, -9.3888) projected
  line L328 (-7.8311, -9.3888) -> (-7.8013, -9.8343) projected
  line L329 (-7.8013, -9.8343) -> (-7.7656, -10.1735) projected
  line L330 (-7.7656, -10.1735) -> (-5.8492, -11.1472) projected
  line L331 (-5.8492, -11.1472) -> (-5.5542, -10.9761) projected
  line L332 (-5.5542, -10.9761) -> (-5.1768, -10.7375) projected
  line L333 (-5.1768, -10.7375) -> (-4.8185, -10.4872) projected
  line L334 (-4.8185, -10.4872) -> (-4.48, -10.2258) projected
  line L335 (-4.48, -10.2258) -> (-4.1624, -9.9537) projected
  line L336 (-4.1624, -9.9537) -> (-3.867, -9.6711) projected
  line L337 (-3.867, -9.6711) -> (-3.5955, -9.3782) projected
  line L338 (-3.5955, -9.3782) -> (-3.3502, -9.0751) projected
  line L339 (-3.3502, -9.0751) -> (-3.1354, -8.7611) projected
  line L340 (-3.1354, -8.7611) -> (-2.9609, -8.4338) projected
  line L341 (-2.9609, -8.4338) -> (-2.8467, -8.0877) projected
  line L342 (-2.8467, -8.0877) -> (-2.7039, -7.7505) projected
  line L343 (-2.7039, -7.7505) -> (-2.615, -7.5871) projected
  line L344 (-2.615, -7.5871) -> (-2.5117, -7.4278) projected
  line L345 (-2.5117, -7.4278) -> (-2.3901, -7.2737) projected
  line L346 (-2.3901, -7.2737) -> (-2.2438, -7.1261) projected
  line L347 (-2.2438, -7.1261) -> (-2.1575, -7.0556) projected
  line L348 (-2.1575, -7.0556) -> (-2.0585, -6.9883) projected
  line L349 (-2.0585, -6.9883) -> (-1.9402, -6.9255) projected
  line L350 (-1.9402, -6.9255) -> (-1.7863, -6.8709) projected
  line L351 (-1.7863, -6.8709) -> (-1.4262, -6.8619) projected
  line L352 (-1.4262, -6.8619) -> (-0.6951, -6.9997) projected
  line L353 (-0.6951, -6.9997) -> (0.0429, -7.0929) projected
  line L354 (0.0429, -7.0929) -> (0.3829, -7.2119) projected
  line L355 (0.3829, -7.2119) -> (0.5127, -7.3112) projected
  line L356 (0.5127, -7.3112) -> (0.6059, -7.4072) projected
  line L357 (0.6059, -7.4072) -> (0.6795, -7.5017) projected
  line L358 (0.6795, -7.5017) -> (0.74, -7.5953) projected
  line L359 (0.74, -7.5953) -> (0.834, -7.7806) projected
  line L360 (0.834, -7.7806) -> (0.9024, -7.9646) projected
  line L361 (0.9024, -7.9646) -> (0.9519, -8.1479) projected
  line L362 (0.9519, -8.1479) -> (0.9863, -8.3307) projected
  line L363 (0.9863, -8.3307) -> (1.0187, -8.6955) projected
  line L364 (1.0187, -8.6955) -> (1.0212, -9.0599) projected
  line L365 (1.0212, -9.0599) -> (1.0869, -9.4249) projected
  line L366 (1.0869, -9.4249) -> (1.1949, -9.7897) projected
  line L367 (1.1949, -9.7897) -> (1.3353, -10.1535) projected
  line L368 (1.3353, -10.1535) -> (1.5039, -10.5156) projected
  line L369 (1.5039, -10.5156) -> (1.6983, -10.8752) projected
  line L370 (1.6983, -10.8752) -> (1.9171, -11.2317) projected
  line L371 (1.9171, -11.2317) -> (2.159, -11.5843) projected
  line L372 (2.159, -11.5843) -> (2.4233, -11.9325) projected
  line L373 (2.4233, -11.9325) -> (2.7092, -12.2754) projected
  line L374 (2.7092, -12.2754) -> (2.9375, -12.5288) projected
  line L375 (2.9375, -12.5288) -> (5.0602, -12.1901) projected
  line L376 (5.0602, -12.1901) -> (5.1983, -11.8783) projected
  line L377 (5.1983, -11.8783) -> (5.3633, -11.4634) projected
  line L378 (5.3633, -11.4634) -> (5.5062, -11.0504) projected
  line L379 (5.5062, -11.0504) -> (5.6263, -10.6399) projected
  line L380 (5.6263, -10.6399) -> (5.7233, -10.2331) projected
  line L381 (5.7233, -10.2331) -> (5.7962, -9.8308) projected
  line L382 (5.7962, -9.8308) -> (5.8437, -9.4343) projected
  line L383 (5.8437, -9.4343) -> (5.864, -9.0449) projected
  line L384 (5.864, -9.0449) -> (5.8532, -8.6645) projected
  line L385 (5.8532, -8.6645) -> (5.802, -8.2972) projected
  line L386 (5.802, -8.2972) -> (5.691, -7.9502) projected
  line L387 (5.691, -7.9502) -> (5.6083, -7.5933) projected
  line L388 (5.6083, -7.5933) -> (5.5841, -7.4089) projected
  line L389 (5.5841, -7.4089) -> (5.5741, -7.2193) projected
  line L390 (5.5741, -7.2193) -> (5.5818, -7.0232) projected
  line L391 (5.5818, -7.0232) -> (5.6135, -6.8178) projected
  line L392 (5.6135, -6.8178) -> (5.6419, -6.7101) projected
  line L393 (5.6419, -6.7101) -> (5.6824, -6.5974) projected
  line L394 (5.6824, -6.5974) -> (5.7412, -6.4771) projected
  line L395 (5.7412, -6.4771) -> (5.8336, -6.3424) projected
  line L396 (5.8336, -6.3424) -> (6.1197, -6.1235) projected
  line L397 (6.1197, -6.1235) -> (6.7921, -5.8052) projected
  line L398 (6.7921, -5.8052) -> (7.444, -5.4468) projected
  line L399 (7.444, -5.4468) -> (7.789, -5.3433) projected
  line L400 (7.789, -5.3433) -> (7.9523, -5.3473) projected
  line L401 (7.9523, -5.3473) -> (8.0842, -5.3702) projected
  line L402 (8.0842, -5.3702) -> (25.3405, 4.0009) projected
  line L403 (53, 15.6179) -> (25.3405, 4.0009) projected
  line L404 (53, -9) -> (53, 15.6179) projected
  line L405 (57, -9) -> (53, -9) projected
  point P0 (0, 0)
  point P1 (53.878, -21.3603)
  point P2 (39.3532, 12.2315)
  point P3 (42.0547, -0.4934)
  point P4 (50.8225, -9)
  point P5 (57, -3.8692)
  point P6 (53, -1.936)
  constraints: 16 end point, 12 symmetric about line, 2 midpoint, 2 point on line, 7 other
extrude "Выдавливание7" add sketch "Эскиз7" against normal up to surface (5 mm away) contours L198 L404 L194 L195
sketch "Эскиз8" plane through (0, 0, 5) normal (0, 0, 1) x (1, 0, 0)
  line L0 (44.0249, 7.1187) -> (53, -1.936) projected
  line L1 (53, -1.936) -> (59.0107, -8)
  circle A0 centre (8.3767, 1.5633) radius 1.6 projected
  circle A1 centre (-2.3455, -2.0471) radius 1.6 projected
  circle A2 centre (-5.9559, 8.675) radius 1.6 projected
  circle A3 centre (4.7663, 12.2855) radius 1.6 projected
  circle A4 centre (1.2104, 5.1192) radius 2.5 projected
  line L2 (57, -9) -> (57, 20.778) projected
  line L3 (53, 20.778) -> (57, 20.778) projected
  line L4 (25.3405, 9.161) -> (53, 20.778) projected
  arc A5 (16.1963, 14.3431) -> (25.3405, 9.161) centre (40.8164, 47.1281) ccw projected
  arc A6 (16.1963, 14.3431) -> (-11.1891, 14.3431) centre (2.5036, -3.8906) ccw projected
  line L5 (-11.1891, 14.3431) -> (-11.0924, 14.1698) projected
  line L6 (-11.0924, 14.1698) -> (-10.8798, 13.8428) projected
  line L7 (-10.8798, 13.8428) -> (-10.6476, 13.5415) projected
  line L8 (-10.6476, 13.5415) -> (-10.3902, 13.2744) projected
  line L9 (-10.3902, 13.2744) -> (-10.0964, 13.0589) projected
  line L10 (-10.0964, 13.0589) -> (-9.8198, 12.8188) projected
  line L11 (-9.8198, 12.8188) -> (-9.6918, 12.6838) projected
  line L12 (-9.6918, 12.6838) -> (-9.5723, 12.5363) projected
  line L13 (-9.5723, 12.5363) -> (-9.4633, 12.3731) projected
  line L14 (-9.4633, 12.3731) -> (-9.3681, 12.1883) projected
  line L15 (-9.3681, 12.1883) -> (-9.3278, 12.0845) projected
  line L16 (-9.3278, 12.0845) -> (-9.2943, 11.9695) projected
  line L17 (-9.2943, 11.9695) -> (-9.2712, 11.8376) projected
  line L18 (-9.2712, 11.8376) -> (-9.2668, 11.6743) projected
  line L19 (-9.2668, 11.6743) -> (-9.3696, 11.329) projected
  line L20 (-9.3696, 11.329) -> (-9.7265, 10.6764) projected
  line L21 (-9.7265, 10.6764) -> (-10.0432, 10.0032) projected
  line L22 (-10.0432, 10.0032) -> (-10.2615, 9.7167) projected
  line L23 (-10.2615, 9.7167) -> (-10.3959, 9.6239) projected
  line L24 (-10.3959, 9.6239) -> (-10.5161, 9.5649) projected
  line L25 (-10.5161, 9.5649) -> (-10.6287, 9.5241) projected
  line L26 (-10.6287, 9.5241) -> (-10.7364, 9.4955) projected
  line L27 (-10.7364, 9.4955) -> (-10.9417, 9.4634) projected
  line L28 (-10.9417, 9.4634) -> (-11.1379, 9.4552) projected
  line L29 (-11.1379, 9.4552) -> (-11.3274, 9.4648) projected
  line L30 (-11.3274, 9.4648) -> (-11.5119, 9.4885) projected
  line L31 (-11.5119, 9.4885) -> (-11.8689, 9.5704) projected
  line L32 (-11.8689, 9.5704) -> (-12.2162, 9.6807) projected
  line L33 (-12.2162, 9.6807) -> (-12.5837, 9.731) projected
  line L34 (-12.5837, 9.731) -> (-12.964, 9.741) projected
  line L35 (-12.964, 9.741) -> (-13.3534, 9.7199) projected
  line L36 (-13.3534, 9.7199) -> (-13.7498, 9.6714) projected
  line L37 (-13.7498, 9.6714) -> (-14.1519, 9.5976) projected
  line L38 (-14.1519, 9.5976) -> (-14.5586, 9.4998) projected
  line L39 (-14.5586, 9.4998) -> (-14.9687, 9.3787) projected
  line L40 (-14.9687, 9.3787) -> (-15.3815, 9.2349) projected
  line L41 (-15.3815, 9.2349) -> (-15.796, 9.069) projected
  line L42 (-15.796, 9.069) -> (-16.1075, 8.9301) projected
  line L43 (-16.1075, 8.9301) -> (-16.4414, 6.8067) projected
  line L44 (-16.4414, 6.8067) -> (-16.1875, 6.579) projected
  line L45 (-16.1875, 6.579) -> (-15.8439, 6.2938) projected
  line L46 (-15.8439, 6.2938) -> (-15.4952, 6.0303) projected
  line L47 (-15.4952, 6.0303) -> (-15.142, 5.7892) projected
  line L48 (-15.142, 5.7892) -> (-14.785, 5.5713) projected
  line L49 (-14.785, 5.5713) -> (-14.425, 5.3776) projected
  line L50 (-14.425, 5.3776) -> (-14.0625, 5.2099) projected
  line L51 (-14.0625, 5.2099) -> (-13.6984, 5.0703) projected
  line L52 (-13.6984, 5.0703) -> (-13.3334, 4.963) projected
  line L53 (-13.3334, 4.963) -> (-12.9682, 4.8982) projected
  line L54 (-12.9682, 4.8982) -> (-12.6038, 4.8965) projected
  line L55 (-12.6038, 4.8965) -> (-12.2389, 4.8649) projected
  line L56 (-12.2389, 4.8649) -> (-12.056, 4.8309) projected
  line L57 (-12.056, 4.8309) -> (-11.8727, 4.7818) projected
  line L58 (-11.8727, 4.7818) -> (-11.6885, 4.7139) projected
  line L59 (-11.6885, 4.7139) -> (-11.5029, 4.6203) projected
  line L60 (-11.5029, 4.6203) -> (-11.4093, 4.56) projected
  line L61 (-11.4093, 4.56) -> (-11.3146, 4.4866) projected
  line L62 (-11.3146, 4.4866) -> (-11.2183, 4.3936) projected
  line L63 (-11.2183, 4.3936) -> (-11.1188, 4.264) projected
  line L64 (-11.1188, 4.264) -> (-10.999, 3.9243) projected
  line L65 (-10.999, 3.9243) -> (-10.9042, 3.1865) projected
  line L66 (-10.9042, 3.1865) -> (-10.7647, 2.4558) projected
  line L67 (-10.7647, 2.4558) -> (-10.7729, 2.0956) projected
  line L68 (-10.7729, 2.0956) -> (-10.8272, 1.9416) projected
  line L69 (-10.8272, 1.9416) -> (-10.8897, 1.8232) projected
  line L70 (-10.8897, 1.8232) -> (-10.9568, 1.724) projected
  line L71 (-10.9568, 1.724) -> (-11.0271, 1.6375) projected
  line L72 (-11.0271, 1.6375) -> (-11.1743, 1.4909) projected
  line L73 (-11.1743, 1.4909) -> (-11.3282, 1.369) projected
  line L74 (-11.3282, 1.369) -> (-11.4872, 1.2653) projected
  line L75 (-11.4872, 1.2653) -> (-11.6504, 1.1761) projected
  line L76 (-11.6504, 1.1761) -> (-11.9874, 1.0325) projected
  line L77 (-11.9874, 1.0325) -> (-12.3332, 0.9175) projected
  line L78 (-12.3332, 0.9175) -> (-12.66, 0.7423) projected
  line L79 (-12.66, 0.7423) -> (-12.9736, 0.5268) projected
  line L80 (-12.9736, 0.5268) -> (-13.2762, 0.2808) projected
  line L81 (-13.2762, 0.2808) -> (-13.5684, 0.0086) projected
  line L82 (-13.5684, 0.0086) -> (-13.8504, -0.2874) projected
  line L83 (-13.8504, -0.2874) -> (-14.1218, -0.6056) projected
  line L84 (-14.1218, -0.6056) -> (-14.3824, -0.9447) projected
  line L85 (-14.3824, -0.9447) -> (-14.6319, -1.3036) projected
  line L86 (-14.6319, -1.3036) -> (-14.8697, -1.6815) projected
  line L87 (-14.8697, -1.6815) -> (-15.0401, -1.9769) projected
  line L88 (-15.0401, -1.9769) -> (-14.0621, -3.891) projected
  line L89 (-14.0621, -3.891) -> (-13.7228, -3.9261) projected
  line L90 (-13.7228, -3.9261) -> (-13.2773, -3.9548) projected
  line L91 (-13.2773, -3.9548) -> (-12.8403, -3.963) projected
  line L92 (-12.8403, -3.963) -> (-12.4128, -3.9505) projected
  line L93 (-12.4128, -3.9505) -> (-11.9959, -3.917) projected
  line L94 (-11.9959, -3.917) -> (-11.5908, -3.862) projected
  line L95 (-11.5908, -3.862) -> (-11.199, -3.7847) projected
  line L96 (-11.199, -3.7847) -> (-10.8224, -3.6836) projected
  line L97 (-10.8224, -3.6836) -> (-10.464, -3.5558) projected
  line L98 (-10.464, -3.5558) -> (-10.1304, -3.3936) projected
  line L99 (-10.1304, -3.3936) -> (-9.8347, -3.1808) projected
  line L100 (-9.8347, -3.1808) -> (-9.5209, -2.9918) projected
  line L101 (-9.5209, -2.9918) -> (-9.353, -2.9118) projected
  line L102 (-9.353, -2.9118) -> (-9.1758, -2.8438) projected
  line L103 (-9.1758, -2.8438) -> (-8.9868, -2.7905) projected
  line L104 (-8.9868, -2.7905) -> (-8.7817, -2.7571) projected
  line L105 (-8.7817, -2.7571) -> (-8.6705, -2.7509) projected
  line L106 (-8.6705, -2.7509) -> (-8.5508, -2.7546) projected
  line L107 (-8.5508, -2.7546) -> (-8.4182, -2.7733) projected
  line L108 (-8.4182, -2.7733) -> (-8.2615, -2.8196) projected
  line L109 (-8.2615, -2.8196) -> (-7.9649, -3.024) projected
  line L110 (-7.9649, -3.024) -> (-7.4545, -3.5652) projected
  line L111 (-7.4545, -3.5652) -> (-6.9122, -4.0744) projected
  line L112 (-6.9122, -4.0744) -> (-6.7071, -4.3705) projected
  line L113 (-6.7071, -4.3705) -> (-6.6604, -4.5271) projected
  line L114 (-6.6604, -4.5271) -> (-6.6415, -4.6596) projected
  line L115 (-6.6415, -4.6596) -> (-6.6374, -4.7793) projected
  line L116 (-6.6374, -4.7793) -> (-6.6435, -4.8906) projected
  line L117 (-6.6435, -4.8906) -> (-6.6764, -5.0958) projected
  line L118 (-6.6764, -5.0958) -> (-6.7292, -5.2848) projected
  line L119 (-6.7292, -5.2848) -> (-6.7969, -5.4622) projected
  line L120 (-6.7969, -5.4622) -> (-6.8765, -5.6303) projected
  line L121 (-6.8765, -5.6303) -> (-7.0647, -5.9445) projected
  line L122 (-7.0647, -5.9445) -> (-7.2769, -6.2407) projected
  line L123 (-7.2769, -6.2407) -> (-7.4384, -6.5746) projected
  line L124 (-7.4384, -6.5746) -> (-7.5654, -6.9333) projected
  line L125 (-7.5654, -6.9333) -> (-7.6656, -7.3102) projected
  line L126 (-7.6656, -7.3102) -> (-7.742, -7.7022) projected
  line L127 (-7.742, -7.7022) -> (-7.7961, -8.1074) projected
  line L128 (-7.7961, -8.1074) -> (-7.8287, -8.5243) projected
  line L129 (-7.8287, -8.5243) -> (-7.8403, -8.9518) projected
  line L130 (-7.8403, -8.9518) -> (-7.8311, -9.3888) projected
  line L131 (-7.8311, -9.3888) -> (-7.8013, -9.8343) projected
  line L132 (-7.8013, -9.8343) -> (-7.7656, -10.1735) projected
  line L133 (-7.7656, -10.1735) -> (-5.8492, -11.1472) projected
  line L134 (-5.8492, -11.1472) -> (-5.5542, -10.9761) projected
  line L135 (-5.5542, -10.9761) -> (-5.1768, -10.7375) projected
  line L136 (-5.1768, -10.7375) -> (-4.8185, -10.4872) projected
  line L137 (-4.8185, -10.4872) -> (-4.48, -10.2258) projected
  line L138 (-4.48, -10.2258) -> (-4.1624, -9.9537) projected
  line L139 (-4.1624, -9.9537) -> (-3.867, -9.6711) projected
  line L140 (-3.867, -9.6711) -> (-3.5955, -9.3782) projected
  line L141 (-3.5955, -9.3782) -> (-3.3502, -9.0751) projected
  line L142 (-3.3502, -9.0751) -> (-3.1354, -8.7611) projected
  line L143 (-3.1354, -8.7611) -> (-2.9609, -8.4338) projected
  line L144 (-2.9609, -8.4338) -> (-2.8467, -8.0877) projected
  line L145 (-2.8467, -8.0877) -> (-2.7039, -7.7505) projected
  line L146 (-2.7039, -7.7505) -> (-2.615, -7.5871) projected
  line L147 (-2.615, -7.5871) -> (-2.5117, -7.4278) projected
  line L148 (-2.5117, -7.4278) -> (-2.3901, -7.2737) projected
  line L149 (-2.3901, -7.2737) -> (-2.2438, -7.1261) projected
  line L150 (-2.2438, -7.1261) -> (-2.1575, -7.0556) projected
  line L151 (-2.1575, -7.0556) -> (-2.0585, -6.9883) projected
  line L152 (-2.0585, -6.9883) -> (-1.9402, -6.9255) projected
  line L153 (-1.9402, -6.9255) -> (-1.7863, -6.8709) projected
  line L154 (-1.7863, -6.8709) -> (-1.4262, -6.8619) projected
  line L155 (-1.4262, -6.8619) -> (-0.6951, -6.9997) projected
  line L156 (-0.6951, -6.9997) -> (0.0429, -7.0929) projected
  line L157 (0.0429, -7.0929) -> (0.3829, -7.2119) projected
  line L158 (0.3829, -7.2119) -> (0.5127, -7.3112) projected
  line L159 (0.5127, -7.3112) -> (0.6059, -7.4072) projected
  line L160 (0.6059, -7.4072) -> (0.6795, -7.5017) projected
  line L161 (0.6795, -7.5017) -> (0.74, -7.5953) projected
  line L162 (0.74, -7.5953) -> (0.834, -7.7806) projected
  line L163 (0.834, -7.7806) -> (0.9024, -7.9646) projected
  line L164 (0.9024, -7.9646) -> (0.9519, -8.1479) projected
  line L165 (0.9519, -8.1479) -> (0.9863, -8.3307) projected
  line L166 (0.9863, -8.3307) -> (1.0187, -8.6955) projected
  line L167 (1.0187, -8.6955) -> (1.0212, -9.0599) projected
  line L168 (1.0212, -9.0599) -> (1.0869, -9.4249) projected
  line L169 (1.0869, -9.4249) -> (1.1949, -9.7897) projected
  line L170 (1.1949, -9.7897) -> (1.3353, -10.1535) projected
  line L171 (1.3353, -10.1535) -> (1.5039, -10.5156) projected
  line L172 (1.5039, -10.5156) -> (1.6983, -10.8752) projected
  line L173 (1.6983, -10.8752) -> (1.9171, -11.2317) projected
  line L174 (1.9171, -11.2317) -> (2.159, -11.5843) projected
  line L175 (2.159, -11.5843) -> (2.4233, -11.9325) projected
  line L176 (2.4233, -11.9325) -> (2.7092, -12.2754) projected
  line L177 (2.7092, -12.2754) -> (2.9375, -12.5288) projected
  line L178 (2.9375, -12.5288) -> (5.0602, -12.1901) projected
  line L179 (5.0602, -12.1901) -> (5.1983, -11.8783) projected
  line L180 (5.1983, -11.8783) -> (5.3633, -11.4634) projected
  line L181 (5.3633, -11.4634) -> (5.5062, -11.0504) projected
  line L182 (5.5062, -11.0504) -> (5.6263, -10.6399) projected
  line L183 (5.6263, -10.6399) -> (5.7233, -10.2331) projected
  line L184 (5.7233, -10.2331) -> (5.7962, -9.8308) projected
  line L185 (5.7962, -9.8308) -> (5.8437, -9.4343) projected
  line L186 (5.8437, -9.4343) -> (5.864, -9.0449) projected
  line L187 (5.864, -9.0449) -> (5.8532, -8.6645) projected
  line L188 (5.8532, -8.6645) -> (5.802, -8.2972) projected
  line L189 (5.802, -8.2972) -> (5.691, -7.9502) projected
  line L190 (5.691, -7.9502) -> (5.6083, -7.5933) projected
  line L191 (5.6083, -7.5933) -> (5.5841, -7.4089) projected
  line L192 (5.5841, -7.4089) -> (5.5741, -7.2193) projected
  line L193 (5.5741, -7.2193) -> (5.5818, -7.0232) projected
  line L194 (5.5818, -7.0232) -> (5.6135, -6.8178) projected
  line L195 (5.6135, -6.8178) -> (5.6419, -6.7101) projected
  line L196 (5.6419, -6.7101) -> (5.6824, -6.5974) projected
  line L197 (5.6824, -6.5974) -> (5.7412, -6.4771) projected
  line L198 (5.7412, -6.4771) -> (5.8336, -6.3424) projected
  line L199 (5.8336, -6.3424) -> (6.1197, -6.1235) projected
  line L200 (6.1197, -6.1235) -> (6.7921, -5.8052) projected
  line L201 (6.7921, -5.8052) -> (7.444, -5.4468) projected
  line L202 (7.444, -5.4468) -> (7.789, -5.3433) projected
  line L203 (7.789, -5.3433) -> (7.9523, -5.3473) projected
  line L204 (7.9523, -5.3473) -> (8.0842, -5.3702) projected
  line L205 (8.0842, -5.3702) -> (25.3405, 4.0009) projected
  line L206 (40.9018, 10.5367) -> (25.3405, 4.0009) projected
  line L207 (40.9018, 10.5367) -> (44.0249, 7.1187) projected
  line L208 (44.0249, 7.1187) -> (53, -1.936) projected
  line L209 (53, -9) -> (53, -1.936) projected
  line L210 (57, -9) -> (53, -9) projected
  point P0 (0, 0)
  point P1 (57, -5.9715)
  constraints: 2 end point
extrude "Выдавливание8" cut sketch "Эскиз8" against normal blind 10 contours L1 L2 L210 L209
